Autodesk Inventor part; units mm, degrees
note: some values were not read from the file. Chosen so that the rebuilt part matches the saved one: direction of "Hole2".
(part 2 of 3)
  spline S48 degree 3 poles (-5.388, 3.5585) (-5.3876, 3.4781) (-5.3714, 3.3993) (-5.3265, 3.291) (-5.3082, 3.2569) (-5.2649, 3.1923) (-5.2385, 3.1606) (-5.1846, 3.1064) (-5.155, 3.0821) (-5.0906, 3.0392) (-5.0541, 3.0199) (-4.9466, 2.9745) (-4.8699, 2.9592) (-4.7883, 2.9589) knots 0 0 0 0 0.25 0.25 0.375 0.375 0.5 0.5 0.625 0.625 0.75 0.75 1 1 1 1
  line L48 (-4.7883, 2.9589) -> (-4.4696, 2.9589)
  spline S49 degree 3 poles (-5.388, 3.5585) (-5.3878, 3.5242) (-5.3848, 3.4901) (-5.379, 3.4568) knots 0 0 0 0 1 1 1 1
  spline S50 degree 3 poles (-5.379, 3.4568) (-5.3755, 3.4426) (-5.3722, 3.4319) (-5.3702, 3.4262) (-5.3698, 3.4252) (-5.3695, 3.4244) (-5.3694, 3.4244) (-5.3693, 3.424) (-5.3691, 3.4237) (-5.369, 3.4236) (-5.369, 3.4235) (-5.369, 3.4235) (-5.369, 3.4235) (-5.3689, 3.4235) (-5.3689, 3.4235) (-5.3689, 3.4235) (-5.3689, 3.4235) (-5.3689, 3.4235) (-5.3689, 3.4235) (-5.3689, 3.4235) (-5.3689, 3.4235) (-5.3689, 3.4236) (-5.3689, 3.4236) (-5.3689, 3.4237) (-5.3689, 3.4238) (-5.369, 3.425) (-5.3696, 3.4282) (-5.3755, 3.4555) (-5.3847, 3.4961) (-5.388, 3.5585) knots 0 0 0 0 0.216458 0.216458 0.250147 0.250147 0.25213 0.25213 0.266562 0.266562 0.270758 0.270758 0.271952 0.271952 0.272738 0.272738 0.27341 0.27341 0.274155 0.274155 0.275353 0.275353 0.277883 0.277883 0.289351 0.289351 0.40678 0.40678 1 1 1 1
  ellipse E4 centre (-4.5542, 3.643) end of major axis (-4.7666, 3.8554) minor radius 0.3 (-4.5538, 3.3429) -> (-4.254, 3.6427) ccw
  ellipse E5 centre (-4.7038, 3.643) end of major axis (-4.4914, 3.8554) minor radius 0.3 (-5.004, 3.6427) -> (-4.7042, 3.3429) ccw
  line L49 (-4.5538, 3.3429) -> (-4.7042, 3.3429)
  spline S51 degree 3 poles (-5.379, 3.4568) (-5.3713, 3.412) (-5.3586, 3.3685) (-5.3265, 3.291) (-5.3082, 3.2569) (-5.2649, 3.1923) (-5.2385, 3.1606) (-5.1846, 3.1064) (-5.155, 3.0821) (-5.0906, 3.0392) (-5.0541, 3.0199) (-4.9466, 2.9745) (-4.8699, 2.9592) (-4.7883, 2.9589) knots 0.106772 0.106772 0.106772 0.106772 0.25 0.25 0.375 0.375 0.5 0.5 0.625 0.625 0.75 0.75 1 1 1 1
  line L50 (-4.7883, 2.9589) -> (-4.4696, 2.9589)
  spline S52 degree 3 poles (-4.4696, 2.9589) (-4.4353, 2.959) (-4.4013, 2.9621) (-4.3679, 2.9678) knots 0 0 0 0 1 1 1 1
  spline S53 degree 3 poles (-4.3679, 2.9678) (-4.3538, 2.9714) (-4.343, 2.9747) (-4.3374, 2.9767) (-4.3363, 2.9771) (-4.3355, 2.9774) (-4.3355, 2.9774) (-4.3351, 2.9776) (-4.3349, 2.9777) (-4.3347, 2.9778) (-4.3347, 2.9779) (-4.3346, 2.9779) (-4.3346, 2.9779) (-4.3346, 2.9779) (-4.3346, 2.9779) (-4.3346, 2.9779) (-4.3346, 2.9779) (-4.3346, 2.9779) (-4.3346, 2.9779) (-4.3347, 2.9779) (-4.3347, 2.9779) (-4.3347, 2.978) (-4.3347, 2.978) (-4.3348, 2.978) (-4.3349, 2.978) (-4.3361, 2.9779) (-4.3393, 2.9772) (-4.3666, 2.9713) (-4.4073, 2.9622) (-4.4696, 2.9589) knots 0 0 0 0 0.216458 0.216458 0.250147 0.250147 0.25213 0.25213 0.266562 0.266562 0.270758 0.270758 0.271952 0.271952 0.272738 0.272738 0.27341 0.27341 0.274155 0.274155 0.275353 0.275353 0.277883 0.277883 0.289351 0.289351 0.40678 0.40678 1 1 1 1
  spline S54 degree 3 poles (-4.3679, 2.9678) (-4.3232, 2.9756) (-4.2796, 2.9882) (-4.2022, 3.0204) (-4.168, 3.0387) (-4.1034, 3.082) (-4.0717, 3.1083) (-4.0175, 3.1623) (-3.9933, 3.1919) (-3.9503, 3.2563) (-3.931, 3.2927) (-3.8857, 3.4003) (-3.8704, 3.4769) (-3.87, 3.5585) knots 0.106772 0.106772 0.106772 0.106772 0.25 0.25 0.375 0.375 0.5 0.5 0.625 0.625 0.75 0.75 1 1 1 1
  arc A17 (1.246, 7.298) -> (-3.254, 7.298) centre (-1.004, 7.298) ccw
  arc A18 (1.246, 7.298) -> (-3.254, 7.298) centre (-1.004, 7.298) ccw
  line L51 (2.4039, 4.698) -> (2.4039, 4.298)
  line L52 (-3.254, 7.298) -> (-3.254, 4.298)
  line L53 (-3.254, 4.298) -> (-3.254, 7.298)
  line L54 (1.246, 4.298) -> (1.246, 7.298)
  line L55 (1.246, 7.298) -> (1.246, 4.298)
  arc A19 (-3.254, 4.298) -> (1.246, 4.298) centre (-1.004, 4.298) ccw
  line L56 (2.4039, 4.698) -> (2.4039, 4.298)
  arc A20 (-3.254, 4.298) -> (1.246, 4.298) centre (-1.004, 4.298) ccw
  spline S55 degree 3 poles (2.4039, 4.298) (2.4039, 4.1157) (2.3896, 3.9357) (2.3611, 3.758) (2.3468, 3.6691) (2.329, 3.5808) (2.3076, 3.4931) (2.2969, 3.4492) (2.2854, 3.4055) (2.2729, 3.3619) (2.2666, 3.3401) (2.2602, 3.3184) (2.2535, 3.2967) (2.2468, 3.275) (2.2403, 3.2545) (2.2328, 3.2316) (2.1123, 2.8657) (1.9342, 2.5291) (1.6997, 2.2234) (1.5825, 2.0705) (1.4542, 1.9295) (1.3149, 1.8001) (1.2452, 1.7355) (1.1728, 1.6738) (1.0976, 1.615) (1.06, 1.5856) (1.0217, 1.557) (0.9828, 1.529) (0.9633, 1.5151) (0.9436, 1.5013) (0.9238, 1.4877) (0.904, 1.4741) (0.8828, 1.46) (0.8638, 1.4475) (0.5591, 1.2478) (0.2306, 1.1007) (-0.1219, 1.0062) knots 0 0 0 0 0.125 0.125 0.125 0.1875 0.1875 0.1875 0.21875 0.21875 0.21875 0.234375 0.234375 0.234375 0.25 0.25 0.25 0.5 0.5 0.5 0.625 0.625 0.625 0.6875 0.6875 0.6875 0.71875 0.71875 0.71875 0.734375 0.734375 0.734375 0.75 0.75 0.75 1 1 1 1
  spline S56 degree 3 poles (5.196, 1.3401) (5.1542, 1.3401) (5.1131, 1.344) (5.0727, 1.3517) (5.0525, 1.3555) (5.0325, 1.3603) (5.0127, 1.3661) (4.9929, 1.3719) (4.9749, 1.3779) (4.9538, 1.3863) (4.8697, 1.4195) (4.7948, 1.4688) (4.7308, 1.5328) (4.6988, 1.5647) (4.6706, 1.5993) (4.6461, 1.6365) (4.6339, 1.6551) (4.6227, 1.6743) (4.6124, 1.6942) (4.6021, 1.7141) (4.592, 1.7364) (4.5843, 1.7558) (4.5536, 1.8333) (4.5381, 1.914) (4.5381, 1.998) knots 0 0 0 0 0.125 0.125 0.125 0.1875 0.1875 0.1875 0.25 0.25 0.25 0.5 0.5 0.5 0.625 0.625 0.625 0.6875 0.6875 0.6875 0.75 0.75 0.75 1 1 1 1
  line L57 (4.5381, 1.998) -> (4.5381, 4.698)
  spline S57 degree 3 poles (5.196, 1.3401) (5.1542, 1.3401) (5.1131, 1.344) (5.0727, 1.3517) (5.0525, 1.3555) (5.0325, 1.3603) (5.0127, 1.3661) (4.9929, 1.3719) (4.9749, 1.3779) (4.9538, 1.3863) (4.8697, 1.4195) (4.7948, 1.4688) (4.7308, 1.5328) (4.6988, 1.5647) (4.6706, 1.5993) (4.6461, 1.6365) (4.6339, 1.6551) (4.6227, 1.6743) (4.6124, 1.6942) (4.6021, 1.7141) (4.592, 1.7364) (4.5843, 1.7558) (4.5536, 1.8333) (4.5381, 1.914) (4.5381, 1.998) knots 0 0 0 0 0.125 0.125 0.125 0.1875 0.1875 0.1875 0.25 0.25 0.25 0.5 0.5 0.5 0.625 0.625 0.625 0.6875 0.6875 0.6875 0.75 0.75 0.75 1 1 1 1
  line L58 (4.5381, 1.998) -> (4.5381, 4.698)
  line L59 (4.1541, 4.698) -> (4.1541, 1.998)
  arc A21 (-0.0226, 0.6353) -> (2.7879, 4.298) centre (-1.004, 4.298) ccw
  spline S58 degree 3 poles (2.4039, 4.298) (2.4039, 4.1157) (2.3896, 3.9357) (2.3611, 3.758) (2.3468, 3.6691) (2.329, 3.5808) (2.3076, 3.4931) (2.2969, 3.4492) (2.2854, 3.4055) (2.2729, 3.3619) (2.2666, 3.3401) (2.2602, 3.3184) (2.2535, 3.2967) (2.2468, 3.275) (2.2403, 3.2545) (2.2328, 3.2316) (2.1123, 2.8657) (1.9342, 2.5291) (1.6997, 2.2234) (1.5825, 2.0705) (1.4542, 1.9295) (1.3149, 1.8001) (1.2452, 1.7355) (1.1728, 1.6738) (1.0976, 1.615) (1.06, 1.5856) (1.0217, 1.557) (0.9828, 1.529) (0.9633, 1.5151) (0.9436, 1.5013) (0.9238, 1.4877) (0.904, 1.4741) (0.8828, 1.46) (0.8638, 1.4475) (0.5591, 1.2478) (0.2306, 1.1007) (-0.1219, 1.0062) knots 0 0 0 0 0.125 0.125 0.125 0.1875 0.1875 0.1875 0.21875 0.21875 0.21875 0.234375 0.234375 0.234375 0.25 0.25 0.25 0.5 0.5 0.5 0.625 0.625 0.625 0.6875 0.6875 0.6875 0.71875 0.71875 0.71875 0.734375 0.734375 0.734375 0.75 0.75 0.75 1 1 1 1
  arc A22 (4.1541, 1.998) -> (5.196, 0.9561) centre (5.196, 1.998) ccw
  arc A23 (9.8138, 0.1517) -> (9.8085, -0.002) centre (12.0442, -0.0022) ccw
  arc A24 (9.8138, 0.1517) -> (9.8085, -0.002) centre (12.0442, -0.0022) ccw
  spline S59 degree 3 poles (9.8085, -0.002) (9.8086, -0.2737) (9.8575, -0.5361) (9.9551, -0.7892) (9.9673, -0.8209) (9.9818, -0.8561) (9.9966, -0.8895) (10.0114, -0.923) (10.0269, -0.9559) (10.0433, -0.9884) (10.0759, -1.0533) (10.1116, -1.1162) (10.1504, -1.1771) (10.228, -1.299) (10.3178, -1.4129) (10.4199, -1.5189) (10.624, -1.7308) (10.8627, -1.8963) (11.1327, -2.012) (11.1665, -2.0264) (11.2, -2.0398) (11.2317, -2.0516) (11.2634, -2.0635) (11.2952, -2.0746) (11.3271, -2.0849) (11.3911, -2.1055) (11.4556, -2.1231) (11.5208, -2.1376) (11.6511, -2.1666) (11.7838, -2.1835) (11.9189, -2.1882) (12.054, -2.1928) (12.1894, -2.1853) (12.3215, -2.1655) (12.4535, -2.1457) (12.5833, -2.1137) (12.7109, -2.0694) (12.8385, -2.0252) (12.9761, -1.9633) (13.1009, -1.8904) (13.2258, -1.8175) (13.3428, -1.7323) (13.4517, -1.6349) (13.5607, -1.5375) (13.661, -1.4285) (13.7478, -1.3127) (13.8346, -1.197) (13.9093, -1.0732) (13.9717, -0.9412) (13.9874, -0.9082) (14.0022, -0.8747) (14.0163, -0.8408) (14.0304, -0.8068) (14.0426, -0.7751) (14.0541, -0.7434) (14.077, -0.6799) (14.0969, -0.6158) (14.1137, -0.5511) (14.1474, -0.4217) (14.1689, -0.2899) (14.1781, -0.1557) knots 0 0 0 0 0.122106 0.122106 0.122106 0.137369 0.137369 0.137369 0.152633 0.152633 0.152633 0.183159 0.183159 0.183159 0.244212 0.244212 0.244212 0.366318 0.366318 0.366318 0.381581 0.381581 0.381581 0.396845 0.396845 0.396845 0.427371 0.427371 0.427371 0.488424 0.488424 0.488424 0.549477 0.549477 0.549477 0.61053 0.61053 0.61053 0.671583 0.671583 0.671583 0.732636 0.732636 0.732636 0.793689 0.793689 0.793689 0.854742 0.854742 0.854742 0.870005 0.870005 0.870005 0.885269 0.885269 0.885269 0.915795 0.915795 0.915795 0.976848 0.976848 0.976848 0.976848
  spline S60 degree 3 poles (9.8085, -0.002) (9.8086, -0.2737) (9.8575, -0.5361) (9.9551, -0.7892) (9.9673, -0.8209) (9.9818, -0.8561) (9.9966, -0.8895) (10.0114, -0.923) (10.0269, -0.9559) (10.0433, -0.9884) (10.0759, -1.0533) (10.1116, -1.1162) (10.1504, -1.1771) (10.228, -1.299) (10.3178, -1.4129) (10.4199, -1.5189) (10.624, -1.7308) (10.8627, -1.8963) (11.1327, -2.012) (11.1665, -2.0264) (11.2, -2.0398) (11.2317, -2.0516) (11.2634, -2.0635) (11.2952, -2.0746) (11.3271, -2.0849) (11.3911, -2.1055) (11.4556, -2.1231) (11.5208, -2.1376) (11.6511, -2.1666) (11.7838, -2.1835) (11.9189, -2.1882) (12.054, -2.1928) (12.1894, -2.1853) (12.3215, -2.1655) (12.4535, -2.1457) (12.5833, -2.1137) (12.7109, -2.0694) (12.8385, -2.0252) (12.9761, -1.9633) (13.1009, -1.8904) (13.2258, -1.8175) (13.3428, -1.7323) (13.4517, -1.6349) (13.5607, -1.5375) (13.661, -1.4285) (13.7478, -1.3127) (13.8346, -1.197) (13.9093, -1.0732) (13.9717, -0.9412) (13.9874, -0.9082) (14.0022, -0.8747) (14.0163, -0.8408) (14.0304, -0.8068) (14.0426, -0.7751) (14.0541, -0.7434) (14.077, -0.6799) (14.0969, -0.6158) (14.1137, -0.5511) (14.1474, -0.4217) (14.1689, -0.2899) (14.1781, -0.1557) knots 0 0 0 0 0.122106 0.122106 0.122106 0.137369 0.137369 0.137369 0.152633 0.152633 0.152633 0.183159 0.183159 0.183159 0.244212 0.244212 0.244212 0.366318 0.366318 0.366318 0.381581 0.381581 0.381581 0.396845 0.396845 0.396845 0.427371 0.427371 0.427371 0.488424 0.488424 0.488424 0.549477 0.549477 0.549477 0.61053 0.61053 0.61053 0.671583 0.671583 0.671583 0.732636 0.732636 0.732636 0.793689 0.793689 0.793689 0.854742 0.854742 0.854742 0.870005 0.870005 0.870005 0.885269 0.885269 0.885269 0.915795 0.915795 0.915795 0.976848 0.976848 0.976848 0.976848
  arc A25 (14.1781, -0.1557) -> (14.1835, -0.002) centre (11.9808, -0.0023) ccw
  spline S61 degree 3 poles (14.1835, -0.002) (14.1834, 0.2697) (14.1346, 0.5321) (14.0369, 0.7852) (14.0247, 0.8168) (14.0102, 0.852) (13.9954, 0.8855) (13.9807, 0.9189) (13.9651, 0.9519) (13.9488, 0.9843) (13.9161, 1.0492) (13.8804, 1.1122) (13.8416, 1.1731) (13.7641, 1.295) (13.6742, 1.4089) (13.5722, 1.5148) (13.368, 1.7268) (13.1293, 1.8922) (12.8593, 2.0079) (12.8255, 2.0224) (12.792, 2.0358) (12.7603, 2.0476) (12.7287, 2.0595) (12.6968, 2.0705) (12.6649, 2.0808) (12.6009, 2.1015) (12.5364, 2.119) (12.4712, 2.1336) (12.341, 2.1626) (12.2082, 2.1795) (12.0731, 2.1841) (11.938, 2.1888) (11.8026, 2.1812) (11.6705, 2.1614) (11.5385, 2.1417) (11.4087, 2.1096) (11.2811, 2.0654) (11.1536, 2.0212) (11.016, 1.9593) (10.8911, 1.8864) (10.7662, 1.8135) (10.6493, 1.7283) (10.5403, 1.6309) (10.4313, 1.5334) (10.331, 1.4245) (10.2442, 1.3087) (10.1574, 1.193) (10.0828, 1.0691) (10.0203, 0.9372) (10.0047, 0.9042) (9.9898, 0.8707) (9.9757, 0.8367) (9.9616, 0.8027) (9.9494, 0.7711) (9.9379, 0.7393) (9.915, 0.6758) (9.8951, 0.6118) (9.8783, 0.5471) (9.8446, 0.4177) (9.8231, 0.2859) (9.8138, 0.1517) knots 0 0 0 0 0.122106 0.122106 0.122106 0.137369 0.137369 0.137369 0.152633 0.152633 0.152633 0.183159 0.183159 0.183159 0.244212 0.244212 0.244212 0.366318 0.366318 0.366318 0.381581 0.381581 0.381581 0.396845 0.396845 0.396845 0.427371 0.427371 0.427371 0.488424 0.488424 0.488424 0.549477 0.549477 0.549477 0.61053 0.61053 0.61053 0.671583 0.671583 0.671583 0.732636 0.732636 0.732636 0.793689 0.793689 0.793689 0.854742 0.854742 0.854742 0.870005 0.870005 0.870005 0.885269 0.885269 0.885269 0.915795 0.915795 0.915795 0.976848 0.976848 0.976848 0.976848
  spline S62 degree 3 poles (14.1835, -0.002) (14.1834, 0.2697) (14.1346, 0.5321) (14.0369, 0.7852) (14.0247, 0.8168) (14.0102, 0.852) (13.9954, 0.8855) (13.9807, 0.9189) (13.9651, 0.9519) (13.9488, 0.9843) (13.9161, 1.0492) (13.8804, 1.1122) (13.8416, 1.1731) (13.7641, 1.295) (13.6742, 1.4089) (13.5722, 1.5148) (13.368, 1.7268) (13.1293, 1.8922) (12.8593, 2.0079) (12.8255, 2.0224) (12.792, 2.0358) (12.7603, 2.0476) (12.7287, 2.0595) (12.6968, 2.0705) (12.6649, 2.0808) (12.6009, 2.1015) (12.5364, 2.119) (12.4712, 2.1336) (12.341, 2.1626) (12.2082, 2.1795) (12.0731, 2.1841) (11.938, 2.1888) (11.8026, 2.1812) (11.6705, 2.1614) (11.5385, 2.1417) (11.4087, 2.1096) (11.2811, 2.0654) (11.1536, 2.0212) (11.016, 1.9593) (10.8911, 1.8864) (10.7662, 1.8135) (10.6493, 1.7283) (10.5403, 1.6309) (10.4313, 1.5334) (10.331, 1.4245) (10.2442, 1.3087) (10.1574, 1.193) (10.0828, 1.0691) (10.0203, 0.9372) (10.0047, 0.9042) (9.9898, 0.8707) (9.9757, 0.8367) (9.9616, 0.8027) (9.9494, 0.7711) (9.9379, 0.7393) (9.915, 0.6758) (9.8951, 0.6118) (9.8783, 0.5471) (9.8446, 0.4177) (9.8231, 0.2859) (9.8138, 0.1517) knots 0 0 0 0 0.122106 0.122106 0.122106 0.137369 0.137369 0.137369 0.152633 0.152633 0.152633 0.183159 0.183159 0.183159 0.244212 0.244212 0.244212 0.366318 0.366318 0.366318 0.381581 0.381581 0.381581 0.396845 0.396845 0.396845 0.427371 0.427371 0.427371 0.488424 0.488424 0.488424 0.549477 0.549477 0.549477 0.61053 0.61053 0.61053 0.671583 0.671583 0.671583 0.732636 0.732636 0.732636 0.793689 0.793689 0.793689 0.854742 0.854742 0.854742 0.870005 0.870005 0.870005 0.885269 0.885269 0.885269 0.915795 0.915795 0.915795 0.976848 0.976848 0.976848 0.976848
  arc A26 (14.1781, -0.1557) -> (14.1835, -0.002) centre (11.9808, -0.0023) ccw
  arc A27 (-3.3692, 1.8445) -> (-1.886, 1.0062) centre (-1.004, 4.298) ccw
  spline S63 degree 3 poles (-3.3692, 1.8445) (-3.4688, 1.9404) (-3.5874, 1.9982) (-3.724, 2.0179) (-3.8605, 2.0375) (-3.9909, 2.0148) (-4.1131, 1.9509) (-4.2353, 1.8869) (-4.3278, 1.7922) (-4.3894, 1.6688) (-4.4511, 1.5454) (-4.4708, 1.4153) (-4.4485, 1.2784) knots 0 0 0 0 0.25 0.25 0.25 0.5 0.5 0.5 0.75 0.75 0.75 1 1 1 1
  arc A28 (-3.6357, 1.5681) -> (-1.9854, 0.6353) centre (-1.004, 4.298) ccw
  arc A29 (-3.6357, 1.5681) -> (-4.0696, 1.3405) centre (-3.8149, 1.3822) ccw
  arc A30 (-2.0872, -2.5435) -> (-1.6459, -2.3617) centre (-1.904, -2.3617) ccw
  line L60 (-1.2619, -2.3617) -> (-1.2619, 0.1928)
  line L61 (-1.2619, -2.3617) -> (-1.2619, 0.1928)
  arc A31 (-1.6459, 0.1928) -> (-1.9854, 0.6353) centre (-2.104, 0.1928) ccw
  spline S64 degree 3 poles (-1.2619, 0.1928) (-1.2619, 0.2378) (-1.2655, 0.2823) (-1.2725, 0.3262) (-1.276, 0.3482) (-1.2805, 0.37) (-1.2857, 0.3917) (-1.291, 0.4134) (-1.2968, 0.4337) (-1.3042, 0.4563) (-1.3338, 0.5465) (-1.3782, 0.6301) (-1.4359, 0.7054) (-1.4648, 0.7431) (-1.4964, 0.7779) (-1.5309, 0.8099) (-1.5481, 0.8259) (-1.566, 0.8411) (-1.5846, 0.8557) (-1.6032, 0.8702) (-1.6237, 0.8848) (-1.6425, 0.8972) (-1.7175, 0.9464) (-1.7987, 0.9827) (-1.886, 1.0062) knots 0 0 0 0 0.125 0.125 0.125 0.1875 0.1875 0.1875 0.25 0.25 0.25 0.5 0.5 0.5 0.625 0.625 0.625 0.6875 0.6875 0.6875 0.75 0.75 0.75 1 1 1 1
  spline S65 degree 3 poles (-1.2619, 0.1928) (-1.2619, 0.2378) (-1.2655, 0.2823) (-1.2725, 0.3262) (-1.276, 0.3482) (-1.2805, 0.37) (-1.2857, 0.3917) (-1.291, 0.4134) (-1.2968, 0.4337) (-1.3042, 0.4563) (-1.3338, 0.5465) (-1.3782, 0.6301) (-1.4359, 0.7054) (-1.4648, 0.7431) (-1.4964, 0.7779) (-1.5309, 0.8099) (-1.5481, 0.8259) (-1.566, 0.8411) (-1.5846, 0.8557) (-1.6032, 0.8702) (-1.6237, 0.8848) (-1.6425, 0.8972) (-1.7175, 0.9464) (-1.7987, 0.9827) (-1.886, 1.0062) knots 0 0 0 0 0.125 0.125 0.125 0.1875 0.1875 0.1875 0.25 0.25 0.25 0.5 0.5 0.5 0.625 0.625 0.625 0.6875 0.6875 0.6875 0.75 0.75 0.75 1 1 1 1
  arc A32 (-3.3692, 1.8445) -> (-1.886, 1.0062) centre (-1.004, 4.298) ccw
  arc A33 (-4.0696, 1.3405) -> (-2.0872, -2.5435) centre (2.9943, 2.498) ccw
  spline S66 degree 3 poles (-3.3692, 1.8445) (-3.4688, 1.9404) (-3.5874, 1.9982) (-3.724, 2.0179) (-3.8605, 2.0375) (-3.9909, 2.0148) (-4.1131, 1.9509) (-4.2353, 1.8869) (-4.3278, 1.7922) (-4.3894, 1.6688) (-4.4511, 1.5454) (-4.4708, 1.4153) (-4.4485, 1.2784) knots 0 0 0 0 0.25 0.25 0.25 0.5 0.5 0.5 0.75 0.75 0.75 1 1 1 1
  spline S67 degree 3 poles (-4.4485, 1.2784) (-4.3216, 0.5044) (-4.0797, -0.2323) (-3.7234, -0.9307) (-3.367, -1.629) (-2.9125, -2.2568) (-2.3598, -2.8139) knots 0 0 0 0 0.5 0.5 0.5 1 1 1 1
  spline S68 degree 3 poles (-4.4485, 1.2784) (-4.3216, 0.5044) (-4.0797, -0.2323) (-3.7234, -0.9307) (-3.367, -1.629) (-2.9125, -2.2568) (-2.3598, -2.8139) knots 0 0 0 0 0.5 0.5 0.5 1 1 1 1
  line L62 (-1.6459, -2.3617) -> (-1.6459, 0.1928)
  line L63 (6.996, 1.3401) -> (5.196, 1.3401)
  line L64 (7.8381, -4.202) -> (7.8381, 0.498)
  line L65 (2.9943, -5.0441) -> (6.996, -5.0441)
  spline S69 degree 3 poles (7.8381, 0.498) (7.8381, 0.5515) (7.8331, 0.6041) (7.8233, 0.6558) (7.8183, 0.6816) (7.8122, 0.7072) (7.8048, 0.7326) (7.7974, 0.7579) (7.7896, 0.781) (7.779, 0.8079) (7.7364, 0.9157) (7.6734, 1.0114) (7.5915, 1.0934) (7.5505, 1.1344) (7.5062, 1.1706) (7.4586, 1.2018) (7.4349, 1.2174) (7.4102, 1.2318) (7.3848, 1.245) (7.3721, 1.2516) (7.3591, 1.2579) (7.346, 1.2639) (7.3329, 1.2699) (7.3184, 1.276) (7.306, 1.2809) (7.2068, 1.3203) (7.1034, 1.34) (6.996, 1.3401) knots 0 0 0 0 0.125 0.125 0.125 0.1875 0.1875 0.1875 0.25 0.25 0.25 0.5 0.5 0.5 0.625 0.625 0.625 0.6875 0.6875 0.6875 0.71875 0.71875 0.71875 0.75 0.75 0.75 1 1 1 1
  spline S70 degree 3 poles (7.8381, 0.498) (7.8381, 0.5515) (7.8331, 0.6041) (7.8233, 0.6558) (7.8183, 0.6816) (7.8122, 0.7072) (7.8048, 0.7326) (7.7974, 0.7579) (7.7896, 0.781) (7.779, 0.8079) (7.7364, 0.9157) (7.6734, 1.0114) (7.5915, 1.0934) (7.5505, 1.1344) (7.5062, 1.1706) (7.4586, 1.2018) (7.4349, 1.2174) (7.4102, 1.2318) (7.3848, 1.245) (7.3721, 1.2516) (7.3591, 1.2579) (7.346, 1.2639) (7.3329, 1.2699) (7.3184, 1.276) (7.306, 1.2809) (7.2068, 1.3203) (7.1034, 1.34) (6.996, 1.3401) knots 0 0 0 0 0.125 0.125 0.125 0.1875 0.1875 0.1875 0.25 0.25 0.25 0.5 0.5 0.5 0.625 0.625 0.625 0.6875 0.6875 0.6875 0.71875 0.71875 0.71875 0.75 0.75 0.75 1 1 1 1
  arc A34 (7.4541, 0.498) -> (6.996, 0.9561) centre (6.996, 0.498) ccw
  line L66 (7.8381, -4.202) -> (7.8381, 0.498)
  line L67 (7.4541, 0.498) -> (7.4541, -4.202)
  line L68 (6.996, 1.3401) -> (5.196, 1.3401)
  line L69 (5.196, 0.9561) -> (6.996, 0.9561)
  spline S71 degree 3 poles (6.996, -5.0441) (7.0495, -5.0441) (7.1021, -5.0391) (7.1538, -5.0293) (7.1796, -5.0243) (7.2052, -5.0182) (7.2306, -5.0108) (7.256, -5.0034) (7.279, -4.9956) (7.306, -4.985) (7.4138, -4.9424) (7.5094, -4.8794) (7.5914, -4.7975) (7.6325, -4.7565) (7.6686, -4.7122) (7.6998, -4.6647) (7.7155, -4.6409) (7.7299, -4.6162) (7.7431, -4.5908) (7.7497, -4.5781) (7.7559, -4.5651) (7.7619, -4.552) (7.7679, -4.5389) (7.774, -4.5244) (7.779, -4.512) (7.8183, -4.4128) (7.838, -4.3094) (7.8381, -4.202) knots 0 0 0 0 0.125 0.125 0.125 0.1875 0.1875 0.1875 0.25 0.25 0.25 0.5 0.5 0.5 0.625 0.625 0.625 0.6875 0.6875 0.6875 0.71875 0.71875 0.71875 0.75 0.75 0.75 1 1 1 1
  spline S72 degree 3 poles (6.996, -5.0441) (7.0495, -5.0441) (7.1021, -5.0391) (7.1538, -5.0293) (7.1796, -5.0243) (7.2052, -5.0182) (7.2306, -5.0108) (7.256, -5.0034) (7.279, -4.9956) (7.306, -4.985) (7.4138, -4.9424) (7.5094, -4.8794) (7.5914, -4.7975) (7.6325, -4.7565) (7.6686, -4.7122) (7.6998, -4.6647) (7.7155, -4.6409) (7.7299, -4.6162) (7.7431, -4.5908) (7.7497, -4.5781) (7.7559, -4.5651) (7.7619, -4.552) (7.7679, -4.5389) (7.774, -4.5244) (7.779, -4.512) (7.8183, -4.4128) (7.838, -4.3094) (7.8381, -4.202) knots 0 0 0 0 0.125 0.125 0.125 0.1875 0.1875 0.1875 0.25 0.25 0.25 0.5 0.5 0.5 0.625 0.625 0.625 0.6875 0.6875 0.6875 0.71875 0.71875 0.71875 0.75 0.75 0.75 1 1 1 1
  line L70 (6.996, -4.6601) -> (2.9943, -4.6601)
  line L71 (2.9943, -5.0441) -> (6.996, -5.0441)
  arc A35 (6.996, -4.6601) -> (7.4541, -4.202) centre (6.996, -4.202) ccw
  spline S73 degree 3 poles (-0.1219, 1.0062) (-0.1654, 0.9945) (-0.2075, 0.9796) (-0.2481, 0.9614) (-0.2684, 0.9523) (-0.2883, 0.9424) (-0.3079, 0.9317) (-0.3275, 0.921) (-0.3456, 0.9102) (-0.3655, 0.8972) (-0.4449, 0.8452) (-0.5142, 0.7807) (-0.5721, 0.7054) (-0.601, 0.6678) (-0.6264, 0.6282) (-0.6484, 0.5867) (-0.6593, 0.5659) (-0.6695, 0.5447) (-0.6787, 0.5229) (-0.6879, 0.5012) (-0.6968, 0.4776) (-0.7038, 0.4563) (-0.7319, 0.3711) (-0.746, 0.2832) (-0.7461, 0.1928) knots 0 0 0 0 0.125 0.125 0.125 0.1875 0.1875 0.1875 0.25 0.25 0.25 0.5 0.5 0.5 0.625 0.625 0.625 0.6875 0.6875 0.6875 0.75 0.75 0.75 1 1 1 1
  spline S74 degree 3 poles (-0.1219, 1.0062) (-0.1654, 0.9945) (-0.2075, 0.9796) (-0.2481, 0.9614) (-0.2684, 0.9523) (-0.2883, 0.9424) (-0.3079, 0.9317) (-0.3275, 0.921) (-0.3456, 0.9102) (-0.3655, 0.8972) (-0.4449, 0.8452) (-0.5142, 0.7807) (-0.5721, 0.7054) (-0.601, 0.6678) (-0.6264, 0.6282) (-0.6484, 0.5867) (-0.6593, 0.5659) (-0.6695, 0.5447) (-0.6787, 0.5229) (-0.6879, 0.5012) (-0.6968, 0.4776) (-0.7038, 0.4563) (-0.7319, 0.3711) (-0.746, 0.2832) (-0.7461, 0.1928) knots 0 0 0 0 0.125 0.125 0.125 0.1875 0.1875 0.1875 0.25 0.25 0.25 0.5 0.5 0.5 0.625 0.625 0.625 0.6875 0.6875 0.6875 0.75 0.75 0.75 1 1 1 1
  spline S75 degree 3 poles (-2.3598, -2.8139) (-2.2681, -2.9061) (-2.1582, -2.9653) (-2.0311, -2.991) (-1.904, -3.0167) (-1.7794, -3.0047) (-1.6595, -2.9553) (-1.5395, -2.906) (-1.4427, -2.8267) (-1.3705, -2.7189) (-1.2983, -2.6112) (-1.262, -2.4921) (-1.2619, -2.3617) knots 0 0 0 0 0.25 0.25 0.25 0.5 0.5 0.5 0.75 0.75 0.75 1 1 1 1
  spline S76 degree 3 poles (-2.3598, -2.8139) (-2.2681, -2.9061) (-2.1582, -2.9653) (-2.0311, -2.991) (-1.904, -3.0167) (-1.7794, -3.0047) (-1.6595, -2.9553) (-1.5395, -2.906) (-1.4427, -2.8267) (-1.3705, -2.7189) (-1.2983, -2.6112) (-1.262, -2.4921) (-1.2619, -2.3617) knots 0 0 0 0 0.25 0.25 0.25 0.5 0.5 0.5 0.75 0.75 0.75 1 1 1 1
  arc A36 (-0.1022, -3.9557) -> (2.9943, -4.6601) centre (2.9943, 2.498) ccw
  line L72 (-0.7461, 0.1928) -> (-0.7461, -3.5427)
  line L73 (-0.7461, 0.1928) -> (-0.7461, -3.5427)
  arc A37 (-0.0226, 0.6353) -> (-0.3621, 0.1928) centre (0.096, 0.1928) ccw
  line L74 (-0.3621, 0.1928) -> (-0.3621, -3.5427)
  ellipse E6 centre (3.0015, 2.5035) end of major axis (-3.3702, -3.8682) minor radius 9 (-6.004, 2.4925) -> (2.9905, -6.502) ccw
  ellipse E7 centre (3.0015, 2.5035) end of major axis (-3.3702, -3.8682) minor radius 9 (-6.004, 2.4925) -> (2.9905, -6.502) ccw
  arc A38 (-0.3621, -3.5427) -> (-0.1022, -3.9557) centre (0.096, -3.5427) ccw
  spline S77 degree 3 poles (-0.7461, -3.5427) (-0.746, -3.7046) (-0.7027, -3.8544) (-0.6167, -3.9912) (-0.5307, -4.128) (-0.4145, -4.2316) (-0.2683, -4.3019) knots 0 0 0 0 0.5 0.5 0.5 1 1 1 1
  spline S78 degree 3 poles (-0.7461, -3.5427) (-0.746, -3.7046) (-0.7027, -3.8544) (-0.6167, -3.9912) (-0.5307, -4.128) (-0.4145, -4.2316) (-0.2683, -4.3019) knots 0 0 0 0 0.5 0.5 0.5 1 1 1 1
  ellipse E8 centre (3.0305, 2.6753) end of major axis (4.5717, 10.243) minor radius 7.6313 (-0.2683, -4.3019) -> (2.9943, -5.0441) ccw
  ellipse E9 centre (3.0305, 2.6753) end of major axis (4.5717, 10.243) minor radius 7.6313 (-0.2683, -4.3019) -> (2.9943, -5.0441) ccw
  arc A39 (-1.9854, 10.9607) -> (-1.6459, 11.4032) centre (-2.104, 11.4032) ccw
  spline S79 degree 3 poles (-1.886, 10.5898) (-1.8425, 10.6015) (-1.8005, 10.6164) (-1.7599, 10.6346) (-1.7396, 10.6436) (-1.7197, 10.6535) (-1.7001, 10.6643) (-1.6805, 10.675) (-1.6623, 10.6858) (-1.6425, 10.6988) (-1.563, 10.7508) (-1.4938, 10.8153) (-1.4359, 10.8905) (-1.407, 10.9282) (-1.3816, 10.9678) (-1.3596, 11.0093) (-1.3486, 11.03) (-1.3385, 11.0513) (-1.3293, 11.073) (-1.3201, 11.0948) (-1.3112, 11.1184) (-1.3042, 11.1397) (-1.2761, 11.2249) (-1.262, 11.3127) (-1.2619, 11.4032) knots 0 0 0 0 0.125 0.125 0.125 0.1875 0.1875 0.1875 0.25 0.25 0.25 0.5 0.5 0.5 0.625 0.625 0.625 0.6875 0.6875 0.6875 0.75 0.75 0.75 1 1 1 1
  arc A40 (-1.9854, 10.9607) -> (-3.7192, 9.9449) centre (-1.004, 7.298) ccw
  spline S80 degree 3 poles (-3.4442, 9.6769) (-3.2303, 9.8963) (-2.9908, 10.0836) (-2.7267, 10.2384) (-2.4626, 10.3932) (-2.1824, 10.5103) (-1.886, 10.5898) knots 0 0 0 0 0.5 0.5 0.5 1 1 1 1
  spline S81 degree 3 poles (-3.4442, 9.6769) (-3.2303, 9.8963) (-2.9908, 10.0836) (-2.7267, 10.2384) (-2.4626, 10.3932) (-2.1824, 10.5103) (-1.886, 10.5898) knots 0 0 0 0 0.5 0.5 0.5 1 1 1 1
  arc A41 (-4.1621, 10.1251) -> (-3.7192, 9.9449) centre (-3.904, 10.1251) ccw
  spline S82 degree 3 poles (-4.5461, 10.1251) (-4.546, 9.9945) (-4.5093, 9.8748) (-4.4367, 9.7667) (-4.3641, 9.6586) (-4.2665, 9.5795) (-4.1459, 9.5303) (-4.0253, 9.4812) (-3.9002, 9.4701) (-3.7727, 9.4966) (-3.6452, 9.5231) (-3.5357, 9.5832) (-3.4442, 9.6769) knots 0 0 0 0 0.25 0.25 0.25 0.5 0.5 0.5 0.75 0.75 0.75 1 1 1 1
  spline S83 degree 3 poles (-4.5461, 10.1251) (-4.546, 9.9945) (-4.5093, 9.8748) (-4.4367, 9.7667) (-4.3641, 9.6586) (-4.2665, 9.5795) (-4.1459, 9.5303) (-4.0253, 9.4812) (-3.9002, 9.4701) (-3.7727, 9.4966) (-3.6452, 9.5231) (-3.5357, 9.5832) (-3.4442, 9.6769) knots 0 0 0 0 0.25 0.25 0.25 0.5 0.5 0.5 0.75 0.75 0.75 1 1 1 1
  arc A42 (-0.3621, 36.8032) -> (-0.0226, 36.3607) centre (0.096, 36.8032) ccw
  spline S84 degree 3 poles (-1.886, 35.9898) (-1.8425, 36.0015) (-1.8005, 36.0164) (-1.7599, 36.0346) (-1.7396, 36.0437) (-1.7197, 36.0536) (-1.7001, 36.0643) (-1.6805, 36.075) (-1.6623, 36.0858) (-1.6425, 36.0988) (-1.563, 36.1508) (-1.4938, 36.2153) (-1.4359, 36.2905) (-1.407, 36.3282) (-1.3816, 36.3678) (-1.3596, 36.4093) (-1.3486, 36.43) (-1.3385, 36.4513) (-1.3293, 36.473) (-1.3201, 36.4948) (-1.3112, 36.5184) (-1.3042, 36.5397) (-1.2761, 36.6249) (-1.262, 36.7127) (-1.2619, 36.8032) knots 0 0 0 0 0.125 0.125 0.125 0.1875 0.1875 0.1875 0.25 0.25 0.25 0.5 0.5 0.5 0.625 0.625 0.625 0.6875 0.6875 0.6875 0.75 0.75 0.75 1 1 1 1
  spline S85 degree 3 poles (-1.886, 35.9898) (-1.8425, 36.0015) (-1.8005, 36.0164) (-1.7599, 36.0346) (-1.7396, 36.0437) (-1.7197, 36.0536) (-1.7001, 36.0643) (-1.6805, 36.075) (-1.6623, 36.0858) (-1.6425, 36.0988) (-1.563, 36.1508) (-1.4938, 36.2153) (-1.4359, 36.2905) (-1.407, 36.3282) (-1.3816, 36.3678) (-1.3596, 36.4093) (-1.3486, 36.43) (-1.3385, 36.4513) (-1.3293, 36.473) (-1.3201, 36.4948) (-1.3112, 36.5184) (-1.3042, 36.5397) (-1.2761, 36.6249) (-1.262, 36.7127) (-1.2619, 36.8032) knots 0 0 0 0 0.125 0.125 0.125 0.1875 0.1875 0.1875 0.25 0.25 0.25 0.5 0.5 0.5 0.625 0.625 0.625 0.6875 0.6875 0.6875 0.75 0.75 0.75 1 1 1 1
  arc A43 (-1.9854, 36.3607) -> (-1.6459, 36.8032) centre (-2.104, 36.8032) ccw
  arc A44 (-1.886, 35.9898) -> (-3.3692, 35.1515) centre (-1.004, 32.698) ccw
  arc A45 (-1.886, 35.9898) -> (-3.3692, 35.1515) centre (-1.004, 32.698) ccw
  line L75 (-1.2619, 36.8032) -> (-1.2619, 39.3577)
  line L76 (-1.2619, 39.3577) -> (-1.2619, 36.8032)
  arc A46 (-1.9854, 36.3607) -> (-3.6357, 35.4279) centre (-1.004, 32.698) ccw
  line L77 (-1.6459, 36.8032) -> (-1.6459, 39.3577)
  line L78 (-0.7461, 40.5387) -> (-0.7461, 36.8032)
  line L79 (-0.7461, 40.5387) -> (-0.7461, 36.8032)
  arc A47 (-2.0872, 39.5394) -> (-4.0696, 35.6555) centre (2.9943, 34.498) ccw
  spline S86 degree 3 poles (-2.3598, 39.8099) (-2.9122, 39.253) (-3.3669, 38.6249) (-3.7234, 37.9266) (-4.0798, 37.2283) (-4.3215, 36.492) (-4.4485, 35.7175) knots 0 0 0 0 0.5 0.5 0.5 1 1 1 1
  spline S87 degree 3 poles (-2.3598, 39.8099) (-2.9122, 39.253) (-3.3669, 38.6249) (-3.7234, 37.9266) (-4.0798, 37.2283) (-4.3215, 36.492) (-4.4485, 35.7175) knots 0 0 0 0 0.5 0.5 0.5 1 1 1 1
  ellipse E10 centre (3.0015, 34.4925) end of major axis (-3.3702, 40.8642) minor radius 9 (2.9905, 43.498) -> (-6.004, 34.5035) ccw
  ellipse E11 centre (3.0015, 34.4925) end of major axis (9.3732, 28.1208) minor radius 9 (2.9905, 43.498) -> (-6.004, 34.5035) ccw
  line L80 (-0.3621, 40.5387) -> (-0.3621, 36.8032)
  spline S88 degree 3 poles (-0.7461, 36.8032) (-0.746, 36.7581) (-0.7425, 36.7136) (-0.7354, 36.6697) (-0.7319, 36.6478) (-0.7275, 36.626) (-0.7223, 36.6043) (-0.717, 36.5826) (-0.7112, 36.5622) (-0.7038, 36.5397) (-0.6741, 36.4495) (-0.6298, 36.3659) (-0.572, 36.2905) (-0.5432, 36.2529) (-0.5115, 36.2181) (-0.4771, 36.1861) (-0.4599, 36.1702) (-0.442, 36.1549) (-0.4234, 36.1403) (-0.4048, 36.1258) (-0.3843, 36.1111) (-0.3655, 36.0988) (-0.2904, 36.0496) (-0.2093, 36.0132) (-0.1219, 35.9898) knots 0 0 0 0 0.125 0.125 0.125 0.1875 0.1875 0.1875 0.25 0.25 0.25 0.5 0.5 0.5 0.625 0.625 0.625 0.6875 0.6875 0.6875 0.75 0.75 0.75 1 1 1 1
  spline S89 degree 3 poles (-0.7461, 36.8032) (-0.746, 36.7581) (-0.7425, 36.7136) (-0.7354, 36.6697) (-0.7319, 36.6478) (-0.7275, 36.626) (-0.7223, 36.6043) (-0.717, 36.5826) (-0.7112, 36.5622) (-0.7038, 36.5397) (-0.6741, 36.4495) (-0.6298, 36.3659) (-0.572, 36.2905) (-0.5432, 36.2529) (-0.5115, 36.2181) (-0.4771, 36.1861) (-0.4599, 36.1702) (-0.442, 36.1549) (-0.4234, 36.1403) (-0.4048, 36.1258) (-0.3843, 36.1111) (-0.3655, 36.0988) (-0.2904, 36.0496) (-0.2093, 36.0132) (-0.1219, 35.9898) knots 0 0 0 0 0.125 0.125 0.125 0.1875 0.1875 0.1875 0.25 0.25 0.25 0.5 0.5 0.5 0.625 0.625 0.625 0.6875 0.6875 0.6875 0.75 0.75 0.75 1 1 1 1
  line L81 (-5.388, 20.7375) -> (-5.388, 16.2585)
  line L82 (-3.87, 16.2585) -> (-3.87, 20.7375)
  line L83 (-3.254, 19.998) -> (-3.254, 16.998)
  line L84 (-3.254, 16.998) -> (-3.254, 19.998)
  spline S90 degree 3 poles (-3.877, 20.8395) (-3.8803, 20.8538) (-3.8834, 20.8646) (-3.8853, 20.8703) (-3.8857, 20.8713) (-3.886, 20.8721) (-3.886, 20.8722) (-3.8862, 20.8725) (-3.8863, 20.8728) (-3.8864, 20.873) (-3.8864, 20.873) (-3.8865, 20.873) (-3.8865, 20.873) (-3.8865, 20.873) (-3.8865, 20.873) (-3.8865, 20.873) (-3.8865, 20.873) (-3.8865, 20.873) (-3.8865, 20.873) (-3.8865, 20.873) (-3.8865, 20.873) (-3.8865, 20.873) (-3.8865, 20.873) (-3.8866, 20.8729) (-3.8866, 20.8727) (-3.8865, 20.8715) (-3.8859, 20.8683) (-3.8805, 20.8409) (-3.8721, 20.8) (-3.87, 20.7375) knots 0 0 0 0 0.216458 0.216458 0.250147 0.250147 0.25213 0.25213 0.266562 0.266562 0.270758 0.270758 0.271952 0.271952 0.272738 0.272738 0.27341 0.27341 0.274154 0.274154 0.275352 0.275352 0.277883 0.277883 0.289351 0.289351 0.40678 0.40678 1 1 1 1
  spline S91 degree 3 poles (-3.87, 20.7375) (-3.8695, 20.7718) (-3.8719, 20.806) (-3.877, 20.8395) knots 0 0 0 0 1 1 1 1
  ellipse E12 centre (-4.5542, 20.6529) end of major axis (-4.3418, 20.8653) minor radius 0.3 (-4.254, 20.6533) -> (-4.5538, 20.9531) ccw
  ellipse E13 centre (-4.7038, 20.6529) end of major axis (-4.9162, 20.8653) minor radius 0.3 (-4.7042, 20.9531) -> (-5.004, 20.6533) ccw
  line L85 (-4.254, 20.6533) -> (-4.254, 16.3427)
  line L86 (-3.87, 16.2585) -> (-3.87, 20.7375)
  line L87 (-5.004, 16.3427) -> (-5.004, 20.6533)
  line L88 (-5.388, 20.7375) -> (-5.388, 16.2585)
  spline S92 degree 3 poles (-0.1219, 26.4062) (-0.1654, 26.3945) (-0.2075, 26.3796) (-0.2481, 26.3614) (-0.2684, 26.3523) (-0.2883, 26.3424) (-0.3079, 26.3317) (-0.3275, 26.321) (-0.3456, 26.3101) (-0.3655, 26.2972) (-0.4449, 26.2452) (-0.5142, 26.1807) (-0.5721, 26.1054) (-0.601, 26.0678) (-0.6264, 26.0282) (-0.6484, 25.9867) (-0.6593, 25.9659) (-0.6695, 25.9447) (-0.6787, 25.9229) (-0.6879, 25.9012) (-0.6968, 25.8776) (-0.7038, 25.8563) (-0.7319, 25.7711) (-0.746, 25.6832) (-0.7461, 25.5928) knots 0 0 0 0 0.125 0.125 0.125 0.1875 0.1875 0.1875 0.25 0.25 0.25 0.5 0.5 0.5 0.625 0.625 0.625 0.6875 0.6875 0.6875 0.75 0.75 0.75 1 1 1 1
  spline S93 degree 3 poles (-0.1219, 26.4062) (-0.1654, 26.3945) (-0.2075, 26.3796) (-0.2481, 26.3614) (-0.2684, 26.3523) (-0.2883, 26.3424) (-0.3079, 26.3317) (-0.3275, 26.321) (-0.3456, 26.3101) (-0.3655, 26.2972) (-0.4449, 26.2452) (-0.5142, 26.1807) (-0.5721, 26.1054) (-0.601, 26.0678) (-0.6264, 26.0282) (-0.6484, 25.9867) (-0.6593, 25.9659) (-0.6695, 25.9447) (-0.6787, 25.9229) (-0.6879, 25.9012) (-0.6968, 25.8776) (-0.7038, 25.8563) (-0.7319, 25.7711) (-0.746, 25.6832) (-0.7461, 25.5928) knots 0 0 0 0 0.125 0.125 0.125 0.1875 0.1875 0.1875 0.25 0.25 0.25 0.5 0.5 0.5 0.625 0.625 0.625 0.6875 0.6875 0.6875 0.75 0.75 0.75 1 1 1 1
  line L89 (-0.3621, 25.5928) -> (-0.3621, 24.1032)
  spline S94 degree 3 poles (-1.2619, 25.5928) (-1.2619, 25.6378) (-1.2655, 25.6823) (-1.2725, 25.7262) (-1.2761, 25.7482) (-1.2805, 25.77) (-1.2857, 25.7917) (-1.291, 25.8134) (-1.2968, 25.8337) (-1.3042, 25.8563) (-1.3339, 25.9465) (-1.3782, 26.0301) (-1.4359, 26.1054) (-1.4648, 26.1431) (-1.4965, 26.1779) (-1.5309, 26.2098) (-1.5481, 26.2258) (-1.566, 26.2411) (-1.5846, 26.2556) (-1.6032, 26.2702) (-1.6237, 26.2848) (-1.6425, 26.2971) (-1.7175, 26.3463) (-1.7987, 26.3827) (-1.886, 26.4062) knots 0 0 0 0 0.125 0.125 0.125 0.1875 0.1875 0.1875 0.25 0.25 0.25 0.5 0.5 0.5 0.625 0.625 0.625 0.6875 0.6875 0.6875 0.75 0.75 0.75 1 1 1 1
  spline S95 degree 3 poles (-1.2619, 25.5928) (-1.2619, 25.6378) (-1.2655, 25.6823) (-1.2725, 25.7262) (-1.2761, 25.7482) (-1.2805, 25.77) (-1.2857, 25.7917) (-1.291, 25.8134) (-1.2968, 25.8337) (-1.3042, 25.8563) (-1.3339, 25.9465) (-1.3782, 26.0301) (-1.4359, 26.1054) (-1.4648, 26.1431) (-1.4965, 26.1779) (-1.5309, 26.2098) (-1.5481, 26.2258) (-1.566, 26.2411) (-1.5846, 26.2556) (-1.6032, 26.2702) (-1.6237, 26.2848) (-1.6425, 26.2971) (-1.7175, 26.3463) (-1.7987, 26.3827) (-1.886, 26.4062) knots 0 0 0 0 0.125 0.125 0.125 0.1875 0.1875 0.1875 0.25 0.25 0.25 0.5 0.5 0.5 0.625 0.625 0.625 0.6875 0.6875 0.6875 0.75 0.75 0.75 1 1 1 1
  line L90 (-0.7461, 25.5928) -> (-0.7461, 24.1032)
  line L91 (-0.7461, 25.5928) -> (-0.7461, 24.1032)
  arc A48 (-1.6459, 25.5928) -> (-1.9854, 26.0353) centre (-2.104, 25.5928) ccw
  line L92 (-1.2619, 24.1032) -> (-1.2619, 25.5928)
  line L93 (-1.2619, 24.1032) -> (-1.2619, 25.5928)
  line L94 (-1.6459, 24.1032) -> (-1.6459, 25.5928)
  spline S96 degree 3 poles (-1.886, 23.2898) (-1.8425, 23.3015) (-1.8005, 23.3164) (-1.7599, 23.3346) (-1.7396, 23.3436) (-1.7197, 23.3535) (-1.7001, 23.3643) (-1.6805, 23.375) (-1.6623, 23.3858) (-1.6425, 23.3988) (-1.563, 23.4508) (-1.4938, 23.5153) (-1.4359, 23.5905) (-1.407, 23.6282) (-1.3816, 23.6678) (-1.3596, 23.7093) (-1.3486, 23.73) (-1.3385, 23.7513) (-1.3293, 23.773) (-1.3201, 23.7948) (-1.3112, 23.8184) (-1.3042, 23.8397) (-1.2761, 23.9249) (-1.262, 24.0127) (-1.2619, 24.1032) knots 0 0 0 0 0.125 0.125 0.125 0.1875 0.1875 0.1875 0.25 0.25 0.25 0.5 0.5 0.5 0.625 0.625 0.625 0.6875 0.6875 0.6875 0.75 0.75 0.75 1 1 1 1
  spline S97 degree 3 poles (-1.886, 23.2898) (-1.8425, 23.3015) (-1.8005, 23.3164) (-1.7599, 23.3346) (-1.7396, 23.3436) (-1.7197, 23.3535) (-1.7001, 23.3643) (-1.6805, 23.375) (-1.6623, 23.3858) (-1.6425, 23.3988) (-1.563, 23.4508) (-1.4938, 23.5153) (-1.4359, 23.5905) (-1.407, 23.6282) (-1.3816, 23.6678) (-1.3596, 23.7093) (-1.3486, 23.73) (-1.3385, 23.7513) (-1.3293, 23.773) (-1.3201, 23.7948) (-1.3112, 23.8184) (-1.3042, 23.8397) (-1.2761, 23.9249) (-1.262, 24.0127) (-1.2619, 24.1032) knots 0 0 0 0 0.125 0.125 0.125 0.1875 0.1875 0.1875 0.25 0.25 0.25 0.5 0.5 0.5 0.625 0.625 0.625 0.6875 0.6875 0.6875 0.75 0.75 0.75 1 1 1 1
  arc A49 (-1.9854, 23.6607) -> (-1.6459, 24.1032) centre (-2.104, 24.1032) ccw
  arc A50 (-3.7192, 27.051) -> (-1.9854, 26.0353) centre (-1.004, 29.698) ccw
  line L95 (-4.1621, 22.8251) -> (-4.1621, 26.8709)
  line L96 (-4.5461, 26.8709) -> (-4.5461, 22.8251)
  line L97 (-4.5461, 26.8709) -> (-4.5461, 22.8251)
  line L98 (-4.7042, 20.9531) -> (-4.5538, 20.9531)
  spline S98 degree 3 poles (-4.8904, 21.33) (-4.9352, 21.3222) (-4.9788, 21.3094) (-5.0563, 21.2771) (-5.0905, 21.2587) (-5.1551, 21.2152) (-5.1868, 21.1888) (-5.241, 21.1346) (-5.2652, 21.1049) (-5.3081, 21.0403) (-5.3274, 21.0038) (-5.3726, 20.896) (-5.3878, 20.8192) (-5.388, 20.7375) knots 0.106772 0.106772 0.106772 0.106772 0.25 0.25 0.375 0.375 0.5 0.5 0.625 0.625 0.75 0.75 1 1 1 1
  spline S99 degree 3 poles (-4.7883, 21.3371) (-4.8687, 21.3367) (-4.9475, 21.3205) (-5.0558, 21.2756) (-5.09, 21.2573) (-5.1545, 21.214) (-5.1862, 21.1877) (-5.2404, 21.1337) (-5.2647, 21.1041) (-5.3076, 21.0397) (-5.3269, 21.0032) (-5.3723, 20.8957) (-5.3876, 20.819) (-5.388, 20.7375) knots 0 0 0 0 0.25 0.25 0.375 0.375 0.5 0.5 0.625 0.625 0.75 0.75 1 1 1 1
  spline S100 degree 3 poles (-3.87, 20.7375) (-3.8704, 20.8178) (-3.8866, 20.8966) (-3.9315, 21.0049) (-3.9498, 21.0391) (-3.9931, 21.1036) (-4.0194, 21.1354) (-4.0734, 21.1896) (-4.103, 21.2138) (-4.1674, 21.2567) (-4.2038, 21.2761) (-4.3114, 21.3214) (-4.388, 21.3367) (-4.4696, 21.3371) knots 0 0 0 0 0.25 0.25 0.375 0.375 0.5 0.5 0.625 0.625 0.75 0.75 1 1 1 1
  spline S101 degree 3 poles (-3.877, 20.8395) (-3.8849, 20.8843) (-3.8976, 20.9279) (-3.93, 21.0054) (-3.9484, 21.0396) (-3.9919, 21.1042) (-4.0183, 21.1359) (-4.0725, 21.1901) (-4.1021, 21.2144) (-4.1668, 21.2572) (-4.2033, 21.2765) (-4.3111, 21.3217) (-4.3879, 21.3369) (-4.4696, 21.3371) knots 0.106772 0.106772 0.106772 0.106772 0.25 0.25 0.375 0.375 0.5 0.5 0.625 0.625 0.75 0.75 1 1 1 1
  spline S102 degree 3 poles (-4.8904, 21.33) (-4.9046, 21.3268) (-4.9154, 21.3237) (-4.9212, 21.3218) (-4.9222, 21.3214) (-4.923, 21.3211) (-4.9231, 21.3211) (-4.9234, 21.3209) (-4.9237, 21.3208) (-4.9239, 21.3207) (-4.9239, 21.3207) (-4.9239, 21.3206) (-4.9239, 21.3206) (-4.9239, 21.3206) (-4.9239, 21.3206) (-4.9239, 21.3206) (-4.9239, 21.3206) (-4.9239, 21.3206) (-4.9239, 21.3206) (-4.9239, 21.3206) (-4.9239, 21.3206) (-4.9239, 21.3206) (-4.9239, 21.3206) (-4.9238, 21.3205) (-4.9236, 21.3205) (-4.9224, 21.3206) (-4.9192, 21.3212) (-4.8918, 21.3266) (-4.8509, 21.335) (-4.7883, 21.3371) knots 0 0 0 0 0.216458 0.216458 0.250147 0.250147 0.25213 0.25213 0.266562 0.266562 0.270757 0.270757 0.271951 0.271951 0.272738 0.272738 0.27341 0.27341 0.274154 0.274154 0.275352 0.275352 0.277883 0.277883 0.289351 0.289351 0.40678 0.40678 1 1 1 1
  spline S103 degree 3 poles (-4.7883, 21.3371) (-4.8227, 21.3376) (-4.8569, 21.3352) (-4.8904, 21.33) knots 0 0 0 0 1 1 1 1
  line L99 (-4.4696, 21.3371) -> (-4.7883, 21.3371)
  line L100 (-4.4696, 21.3371) -> (-4.7883, 21.3371)
  spline S104 degree 3 poles (-4.5461, 22.8251) (-4.546, 22.6945) (-4.5093, 22.5748) (-4.4367, 22.4667) (-4.3641, 22.3586) (-4.2665, 22.2795) (-4.1459, 22.2303) (-4.0253, 22.1812) (-3.9002, 22.1701) (-3.7727, 22.1966) (-3.6452, 22.2231) (-3.5357, 22.2832) (-3.4442, 22.3769) knots 0 0 0 0 0.25 0.25 0.25 0.5 0.5 0.5 0.75 0.75 0.75 1 1 1 1
  spline S105 degree 3 poles (-4.5461, 22.8251) (-4.546, 22.6945) (-4.5093, 22.5748) (-4.4367, 22.4667) (-4.3641, 22.3586) (-4.2665, 22.2795) (-4.1459, 22.2303) (-4.0253, 22.1812) (-3.9002, 22.1701) (-3.7727, 22.1966) (-3.6452, 22.2231) (-3.5357, 22.2832) (-3.4442, 22.3769) knots 0 0 0 0 0.25 0.25 0.25 0.5 0.5 0.5 0.75 0.75 0.75 1 1 1 1
  arc A51 (-4.1621, 22.8251) -> (-3.7192, 22.6449) centre (-3.904, 22.8251) ccw
  spline S106 degree 3 poles (-3.4442, 22.3769) (-3.2303, 22.5963) (-2.9908, 22.7836) (-2.7267, 22.9384) (-2.4626, 23.0932) (-2.1824, 23.2103) (-1.886, 23.2898) knots 0 0 0 0 0.5 0.5 0.5 1 1 1 1
  spline S107 degree 3 poles (-3.4442, 22.3769) (-3.2303, 22.5963) (-2.9908, 22.7836) (-2.7267, 22.9384) (-2.4626, 23.0932) (-2.1824, 23.2103) (-1.886, 23.2898) knots 0 0 0 0 0.5 0.5 0.5 1 1 1 1
  arc A52 (-1.9854, 23.6607) -> (-3.7192, 22.6449) centre (-1.004, 19.998) ccw
  spline S108 degree 3 poles (-0.7461, 24.1032) (-0.746, 24.0581) (-0.7425, 24.0136) (-0.7354, 23.9697) (-0.7319, 23.9478) (-0.7275, 23.926) (-0.7223, 23.9043) (-0.717, 23.8826) (-0.7112, 23.8622) (-0.7038, 23.8397) (-0.6741, 23.7495) (-0.6298, 23.6659) (-0.572, 23.5905) (-0.5432, 23.5529) (-0.5115, 23.5181) (-0.4771, 23.4861) (-0.4599, 23.4702) (-0.442, 23.4549) (-0.4234, 23.4403) (-0.4048, 23.4258) (-0.3843, 23.4111) (-0.3655, 23.3988) (-0.2904, 23.3496) (-0.2093, 23.3132) (-0.1219, 23.2898) knots 0 0 0 0 0.125 0.125 0.125 0.1875 0.1875 0.1875 0.25 0.25 0.25 0.5 0.5 0.5 0.625 0.625 0.625 0.6875 0.6875 0.6875 0.75 0.75 0.75 1 1 1 1
  spline S109 degree 3 poles (-0.7461, 24.1032) (-0.746, 24.0581) (-0.7425, 24.0136) (-0.7354, 23.9697) (-0.7319, 23.9478) (-0.7275, 23.926) (-0.7223, 23.9043) (-0.717, 23.8826) (-0.7112, 23.8622) (-0.7038, 23.8397) (-0.6741, 23.7495) (-0.6298, 23.6659) (-0.572, 23.5905) (-0.5432, 23.5529) (-0.5115, 23.5181) (-0.4771, 23.4861) (-0.4599, 23.4702) (-0.442, 23.4549) (-0.4234, 23.4403) (-0.4048, 23.4258) (-0.3843, 23.4111) (-0.3655, 23.3988) (-0.2904, 23.3496) (-0.2093, 23.3132) (-0.1219, 23.2898) knots 0 0 0 0 0.125 0.125 0.125 0.1875 0.1875 0.1875 0.25 0.25 0.25 0.5 0.5 0.5 0.625 0.625 0.625 0.6875 0.6875 0.6875 0.75 0.75 0.75 1 1 1 1
  line L101 (2.4039, 19.998) -> (2.4039, 19.598)
  line L102 (2.4039, 19.998) -> (2.4039, 19.598)
  arc A53 (2.7879, 19.598) -> (3.246, 19.1399) centre (3.246, 19.598) ccw
  spline S110 degree 3 poles (2.4039, 19.598) (2.404, 19.5444) (2.4089, 19.4918) (2.4188, 19.4402) (2.4237, 19.4144) (2.4298, 19.3888) (2.4372, 19.3634) (2.4446, 19.338) (2.4524, 19.315) (2.463, 19.288) (2.5057, 19.1802) (2.5687, 19.0846) (2.6506, 19.0025) (2.6915, 18.9615) (2.7358, 18.9254) (2.7834, 18.8942) (2.8072, 18.8785) (2.8318, 18.8641) (2.8572, 18.8509) (2.8699, 18.8443) (2.8829, 18.8381) (2.896, 18.8321) (2.9092, 18.8261) (2.9236, 18.8199) (2.936, 18.815) (3.0353, 18.7757) (3.1386, 18.756) (3.246, 18.7559) knots 0 0 0 0 0.125 0.125 0.125 0.1875 0.1875 0.1875 0.25 0.25 0.25 0.5 0.5 0.5 0.625 0.625 0.625 0.6875 0.6875 0.6875 0.71875 0.71875 0.71875 0.75 0.75 0.75 1 1 1 1
  spline S111 degree 3 poles (2.4039, 19.598) (2.404, 19.5444) (2.4089, 19.4918) (2.4188, 19.4402) (2.4237, 19.4144) (2.4298, 19.3888) (2.4372, 19.3634) (2.4446, 19.338) (2.4524, 19.315) (2.463, 19.288) (2.5057, 19.1802) (2.5687, 19.0846) (2.6506, 19.0025) (2.6915, 18.9615) (2.7358, 18.9254) (2.7834, 18.8942) (2.8072, 18.8785) (2.8318, 18.8641) (2.8572, 18.8509) (2.8699, 18.8443) (2.8829, 18.8381) (2.896, 18.8321) (2.9092, 18.8261) (2.9236, 18.8199) (2.936, 18.815) (3.0353, 18.7757) (3.1386, 18.756) (3.246, 18.7559) knots 0 0 0 0 0.125 0.125 0.125 0.1875 0.1875 0.1875 0.25 0.25 0.25 0.5 0.5 0.5 0.625 0.625 0.625 0.6875 0.6875 0.6875 0.71875 0.71875 0.71875 0.75 0.75 0.75 1 1 1 1
  line L103 (7.4541, 24.498) -> (7.4541, 19.598)
  line L104 (7.8381, 19.598) -> (7.8381, 24.498)
  line L105 (7.8381, 19.598) -> (7.8381, 24.498)
  line L106 (3.246, 19.1399) -> (6.996, 19.1399)
  line L107 (3.246, 18.7559) -> (6.996, 18.7559)
  line L108 (3.246, 18.7559) -> (6.996, 18.7559)
  spline S112 degree 3 poles (6.996, 18.7559) (7.0495, 18.7559) (7.1021, 18.761) (7.1538, 18.7708) (7.1796, 18.7757) (7.2052, 18.7819) (7.2306, 18.7892) (7.256, 18.7966) (7.279, 18.8044) (7.306, 18.815) (7.4138, 18.8577) (7.5094, 18.9206) (7.5914, 19.0026) (7.6324, 19.0435) (7.6684, 19.0879) (7.6997, 19.1354) (7.7153, 19.1592) (7.7298, 19.1838) (7.743, 19.2092) (7.7496, 19.2219) (7.7559, 19.2349) (7.7619, 19.248) (7.7679, 19.2611) (7.7741, 19.2756) (7.779, 19.288) (7.8183, 19.3873) (7.838, 19.4906) (7.8381, 19.598) knots 0 0 0 0 0.125 0.125 0.125 0.1875 0.1875 0.1875 0.25 0.25 0.25 0.5 0.5 0.5 0.625 0.625 0.625 0.6875 0.6875 0.6875 0.71875 0.71875 0.71875 0.75 0.75 0.75 1 1 1 1
  spline S113 degree 3 poles (6.996, 18.7559) (7.0495, 18.7559) (7.1021, 18.761) (7.1538, 18.7708) (7.1796, 18.7757) (7.2052, 18.7819) (7.2306, 18.7892) (7.256, 18.7966) (7.279, 18.8044) (7.306, 18.815) (7.4138, 18.8577) (7.5094, 18.9206) (7.5914, 19.0026) (7.6324, 19.0435) (7.6684, 19.0879) (7.6997, 19.1354) (7.7153, 19.1592) (7.7298, 19.1838) (7.743, 19.2092) (7.7496, 19.2219) (7.7559, 19.2349) (7.7619, 19.248) (7.7679, 19.2611) (7.7741, 19.2756) (7.779, 19.288) (7.8183, 19.3873) (7.838, 19.4906) (7.8381, 19.598) knots 0 0 0 0 0.125 0.125 0.125 0.1875 0.1875 0.1875 0.25 0.25 0.25 0.5 0.5 0.5 0.625 0.625 0.625 0.6875 0.6875 0.6875 0.71875 0.71875 0.71875 0.75 0.75 0.75 1 1 1 1
  arc A54 (6.996, 19.1399) -> (7.4541, 19.598) centre (6.996, 19.598) ccw
  line L109 (1.246, 16.998) -> (1.246, 19.998)
  line L110 (1.246, 19.998) -> (1.246, 16.998)
  spline S114 degree 3 poles (-0.1219, 23.2898) (0.0541, 23.2426) (0.2243, 23.1822) (0.3886, 23.1086) (0.4707, 23.0719) (0.5514, 23.0318) (0.6306, 22.9884) (0.6702, 22.9667) (0.7094, 22.9442) (0.7483, 22.9209) (0.7677, 22.9093) (0.7871, 22.8974) (0.8063, 22.8853) (0.8256, 22.8732) (0.8436, 22.8617) (0.8638, 22.8485) (1.186, 22.6374) (1.4652, 22.3782) (1.6997, 22.0726) (1.817, 21.9198) (1.92, 21.7594) (2.0089, 21.5913) (2.0533, 21.5073) (2.0942, 21.4214) (2.1315, 21.3335) (2.1502, 21.2896) (2.1679, 21.2452) (2.1848, 21.2004) (2.1933, 21.1779) (2.2015, 21.1554) (2.2095, 21.1327) (2.2175, 21.11) (2.2257, 21.086) (2.2328, 21.0643) (2.3468, 20.7184) (2.4039, 20.3629) (2.4039, 19.998) knots 0 0 0 0 0.125 0.125 0.125 0.1875 0.1875 0.1875 0.21875 0.21875 0.21875 0.234375 0.234375 0.234375 0.25 0.25 0.25 0.5 0.5 0.5 0.625 0.625 0.625 0.6875 0.6875 0.6875 0.71875 0.71875 0.71875 0.734375 0.734375 0.734375 0.75 0.75 0.75 1 1 1 1
  arc A55 (1.246, 19.998) -> (-3.254, 19.998) centre (-1.004, 19.998) ccw
  arc A56 (1.246, 19.998) -> (-3.254, 19.998) centre (-1.004, 19.998) ccw
  arc A57 (2.7879, 19.998) -> (-0.0226, 23.6607) centre (-1.004, 19.998) ccw
  spline S115 degree 3 poles (-0.1219, 23.2898) (0.0541, 23.2426) (0.2243, 23.1822) (0.3886, 23.1086) (0.4707, 23.0719) (0.5514, 23.0318) (0.6306, 22.9884) (0.6702, 22.9667) (0.7094, 22.9442) (0.7483, 22.9209) (0.7677, 22.9093) (0.7871, 22.8974) (0.8063, 22.8853) (0.8256, 22.8732) (0.8436, 22.8617) (0.8638, 22.8485) (1.186, 22.6374) (1.4652, 22.3782) (1.6997, 22.0726) (1.817, 21.9198) (1.92, 21.7594) (2.0089, 21.5913) (2.0533, 21.5073) (2.0942, 21.4214) (2.1315, 21.3335) (2.1502, 21.2896) (2.1679, 21.2452) (2.1848, 21.2004) (2.1933, 21.1779) (2.2015, 21.1554) (2.2095, 21.1327) (2.2175, 21.11) (2.2257, 21.086) (2.2328, 21.0643) (2.3468, 20.7184) (2.4039, 20.3629) (2.4039, 19.998) knots 0 0 0 0 0.125 0.125 0.125 0.1875 0.1875 0.1875 0.21875 0.21875 0.21875 0.234375 0.234375 0.234375 0.25 0.25 0.25 0.5 0.5 0.5 0.625 0.625 0.625 0.6875 0.6875 0.6875 0.71875 0.71875 0.71875 0.734375 0.734375 0.734375 0.75 0.75 0.75 1 1 1 1
  line L111 (2.7879, 19.598) -> (2.7879, 19.998)
  arc A58 (-0.3621, 24.1032) -> (-0.0226, 23.6607) centre (0.096, 24.1032) ccw
  arc A59 (7.4541, 24.498) -> (6.996, 24.9561) centre (6.996, 24.498) ccw
  spline S116 degree 3 poles (7.8381, 24.498) (7.8381, 24.5515) (7.8331, 24.6041) (7.8233, 24.6558) (7.8183, 24.6816) (7.8122, 24.7072) (7.8048, 24.7326) (7.7974, 24.7579) (7.7896, 24.781) (7.779, 24.8079) (7.7364, 24.9157) (7.6734, 25.0114) (7.5915, 25.0934) (7.5505, 25.1344) (7.5062, 25.1706) (7.4586, 25.2018) (7.4349, 25.2174) (7.4102, 25.2318) (7.3848, 25.245) (7.3721, 25.2516) (7.3591, 25.2579) (7.346, 25.2639) (7.3329, 25.2699) (7.3184, 25.276) (7.306, 25.2809) (7.2068, 25.3203) (7.1034, 25.34) (6.996, 25.3401) knots 0 0 0 0 0.125 0.125 0.125 0.1875 0.1875 0.1875 0.25 0.25 0.25 0.5 0.5 0.5 0.625 0.625 0.625 0.6875 0.6875 0.6875 0.71875 0.71875 0.71875 0.75 0.75 0.75 1 1 1 1
  spline S117 degree 3 poles (7.8381, 24.498) (7.8381, 24.5515) (7.8331, 24.6041) (7.8233, 24.6558) (7.8183, 24.6816) (7.8122, 24.7072) (7.8048, 24.7326) (7.7974, 24.7579) (7.7896, 24.781) (7.779, 24.8079) (7.7364, 24.9157) (7.6734, 25.0114) (7.5915, 25.0934) (7.5505, 25.1344) (7.5062, 25.1706) (7.4586, 25.2018) (7.4349, 25.2174) (7.4102, 25.2318) (7.3848, 25.245) (7.3721, 25.2516) (7.3591, 25.2579) (7.346, 25.2639) (7.3329, 25.2699) (7.3184, 25.276) (7.306, 25.2809) (7.2068, 25.3203) (7.1034, 25.34) (6.996, 25.3401) knots 0 0 0 0 0.125 0.125 0.125 0.1875 0.1875 0.1875 0.25 0.25 0.25 0.5 0.5 0.5 0.625 0.625 0.625 0.6875 0.6875 0.6875 0.71875 0.71875 0.71875 0.75 0.75 0.75 1 1 1 1
  line L112 (5.196, 24.9561) -> (6.996, 24.9561)
  line L113 (6.996, 25.3401) -> (5.196, 25.3401)
  arc A60 (4.1541, 25.998) -> (5.196, 24.9561) centre (5.196, 25.998) ccw
  spline S118 degree 3 poles (5.196, 25.3401) (5.1542, 25.3401) (5.1131, 25.344) (5.0727, 25.3517) (5.0525, 25.3555) (5.0325, 25.3603) (5.0127, 25.3661) (4.9929, 25.3719) (4.9749, 25.3779) (4.9538, 25.3863) (4.8697, 25.4195) (4.7948, 25.4688) (4.7308, 25.5328) (4.6988, 25.5647) (4.6706, 25.5993) (4.6461, 25.6365) (4.6339, 25.6551) (4.6227, 25.6743) (4.6124, 25.6942) (4.6021, 25.7141) (4.592, 25.7364) (4.5843, 25.7558) (4.5536, 25.8333) (4.5381, 25.914) (4.5381, 25.998) knots 0 0 0 0 0.125 0.125 0.125 0.1875 0.1875 0.1875 0.25 0.25 0.25 0.5 0.5 0.5 0.625 0.625 0.625 0.6875 0.6875 0.6875 0.75 0.75 0.75 1 1 1 1
  spline S119 degree 3 poles (5.196, 25.3401) (5.1542, 25.3401) (5.1131, 25.344) (5.0727, 25.3517) (5.0525, 25.3555) (5.0325, 25.3603) (5.0127, 25.3661) (4.9929, 25.3719) (4.9749, 25.3779) (4.9538, 25.3863) (4.8697, 25.4195) (4.7948, 25.4688) (4.7308, 25.5328) (4.6988, 25.5647) (4.6706, 25.5993) (4.6461, 25.6365) (4.6339, 25.6551) (4.6227, 25.6743) (4.6124, 25.6942) (4.6021, 25.7141) (4.592, 25.7364) (4.5843, 25.7558) (4.5536, 25.8333) (4.5381, 25.914) (4.5381, 25.998) knots 0 0 0 0 0.125 0.125 0.125 0.1875 0.1875 0.1875 0.25 0.25 0.25 0.5 0.5 0.5 0.625 0.625 0.625 0.6875 0.6875 0.6875 0.75 0.75 0.75 1 1 1 1
  line L114 (6.996, 25.3401) -> (5.196, 25.3401)
  arc A61 (-3.7192, 27.051) -> (-4.1621, 26.8709) centre (-3.904, 26.8709) ccw